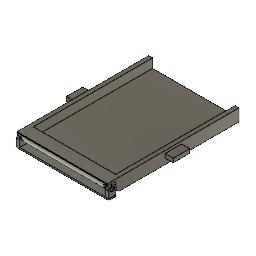
puhelimen paikka tapit ja osat v7 (Autodesk Fusion 360 design; units mm, degrees)
Autodesk Fusion 360 part; units mm, degrees
sketch "Sketch1" plane through (0, 0, 0) normal (0, 0, 1) x (1, 0, 0)
  line L0 (-50, 80) -> (60, 80)
  line L1 (60, 80) -> (60, -80)
  line L2 (60, -80) -> (-50, -80)
  line L3 (-50, -80) -> (-50, 80)
  dimension "d1" = 110
  dimension "d2" = 160
  constraint horizontal L0
  constraint vertical L1
  constraint horizontal L2
  constraint vertical L3
  measures "d1" distance of L0.start L0.end
  measures "d2" distance of L0.start L2.end
extrude "Extrude1" add sketch "Sketch1" along normal blind 12 makes body 1
sketch "Sketch2" plane through (0, 0, 12) normal (0, 0, 1) x (-1, 0, 0)
  line L0 (50, 80) -> (-60, 80)
  line L1 (-60, 80) -> (-60, -80)
  line L2 (-60, -80) -> (50, -80)
  line L3 (50, -80) -> (50, 80)
  line L4 (45, -80) -> (-55, -80)
  line L5 (-55, -80) -> (-55, 70)
  line L6 (-55, 70) -> (45, 70)
  line L7 (45, 70) -> (45, -80)
  constraint horizontal L4
  constraint vertical L5
  constraint horizontal L6
  constraint vertical L7
  constraint coincident L2 L4.start
extrude "Extrude2" cut sketch "Sketch2" against normal blind 10 contours L2 L4 L5 L6 L7 bodies 1
sketch "Sketch3" plane through (0, -70, 0) normal (0, 1, 0) x (-1, 0, 0)
  line L0 (45, 12) -> (-55, 12)
  line L1 (-55, 12) -> (-55, 2)
  line L2 (-55, 2) -> (45, 2)
  line L3 (45, 2) -> (45, 12)
  line L4 (-55, 12) -> (45, 12)
  line L5 (45, 12) -> (45, 11)
  line L6 (45, 11) -> (-55, 11)
  line L7 (-55, 11) -> (-55, 12)
  dimension "d7" = 1
  constraint horizontal L4
  constraint vertical L5
  constraint horizontal L6
  constraint vertical L7
  constraint coincident L0.end L1.start
  measures "d7" distance of L0.end L6.end
extrude "Extrude3" add sketch "Sketch3" along normal blind 5 contours L0 L1 L3 L4 L5 L6 L7 bodies 1
fillet "Fillet1" radius 12 1 edges at (5, -80, 0) on bodies 1
sketch "Sketch4" plane through (60, 0, 0) normal (1, 0, 0) x (0, 1, 0)
  arc A0 (-80, 12) -> (-68, 0) centre (-68, 12) ccw
  line L0 (-68, 0) -> (80, 0)
  line L1 (80, 0) -> (80, 12)
  line L2 (80, 12) -> (-80, 12)
  line L3 (-10, 10) -> (10, 10)
  line L4 (10, 10) -> (10, 5)
  line L5 (10, 5) -> (-10, 5)
  line L6 (-10, 5) -> (-10, 10)
  dimension "d12" = 20
  constraint horizontal L3
  constraint vertical L4
  constraint horizontal L5
  constraint vertical L6
  measures "d12" distance of L3.start L3.end
extrude "Extrude4" add sketch "Sketch4" along normal blind 10 contours L3 L4 L5 L6 bodies 1
sketch "Sketch5" plane through (-50, 0, 0) normal (-1, 0, 0) x (0, -1, 0)
  arc A0 (68, 0) -> (80, 12) centre (68, 12) ccw
  line L0 (80, 12) -> (-80, 12)
  line L1 (-80, 12) -> (-80, 0)
  line L2 (-80, 0) -> (68, 0)
  line L3 (-10, 10) -> (10, 10)
  line L4 (10, 10) -> (10, 5)
  line L5 (10, 5) -> (-10, 5)
  line L6 (-10, 5) -> (-10, 10)
  dimension "d15" = 20
  constraint horizontal L3
  constraint vertical L4
  constraint horizontal L5
  constraint vertical L6
  measures "d15" distance of L3.start L3.end
extrude "Extrude5" add sketch "Sketch5" along normal blind 10 contours L3 L4 L5 L6 bodies 1
extrude "Extrude6" add 2 faces at (-13.3333, -80, 11.9984) (21.6667, -75, 12) along direction (0, 0, 1) blind 1 on bodies 1 bodies 1
extrude "Extrude7" add 1 faces at (-13.3333, -18.6683, 0) along direction (0, 0, -1) blind 2 on bodies 1 bodies 1
fillet "Fillet2" radius 3 1 edges at (5, -68, -2) on bodies 1
sketch "Sketch6" plane through (60, 0, 0) normal (1, 0, 0) x (0, 1, 0)
  arc A0 (-68, 0) -> (-65.1716, -2) centre (-65.1716, 1) ccw
  line L0 (-65.1716, -2) -> (80, -2)
  line L1 (80, -2) -> (80, 13)
  line L2 (80, 13) -> (-80, 13)
  line L3 (-80, 13) -> (-80, 12)
  arc A1 (-80, 12) -> (-68, 0) centre (-68, 12) ccw
  line L4 (-10, 5) -> (-10, 10)
  line L5 (-10, 10) -> (10, 10)
  line L6 (10, 10) -> (10, 5)
  line L7 (10, 5) -> (-10, 5)
  line L8 (-80, 10.5) -> (-70, 10.5)
  line L9 (-70, 10.5) -> (-70, 0)
  line L10 (-70, 0) -> (-80, 0)
  line L11 (-80, 0) -> (-80, 10.5)
  dimension "d24" = 10
  constraint horizontal L8
  constraint vertical L9
  constraint horizontal L10
  constraint vertical L11
  measures "d24" distance of L8.start L8.end
extrude "Extrude8" cut sketch "Sketch6" against normal blind 5 contours A1 L8 L9 bodies 1
sketch "Sketch7" plane through (55, 0, 0) normal (1, 0, 0) x (0, 1, 0)
  arc A0 (-79.9059, 10.5) -> (-70, 0.1678) centre (-68, 12) ccw
  line L0 (-70, 0.1678) -> (-70, 2)
  line L1 (-70, 2) -> (-70, 10.5)
  line L2 (-70, 10.5) -> (-79.9059, 10.5)
  line L3 (-70, 10.5) -> (-75, 10.5)
  line L4 (-75, 10.5) -> (-75, 5.5)
  line L5 (-75, 5.5) -> (-70, 5.5)
  line L6 (-70, 5.5) -> (-70, 10.5)
  circle A1 centre (-75, 5.5) radius 2.25
  dimension "d27" = 5
  dimension "d28" = 5
  dimension "d29" = 4.5
  constraint horizontal L3
  constraint vertical L4
  constraint horizontal L5
  constraint vertical L6
  constraint coincident L1.end L2.start
  constraint coincident L4.end L5.start
  measures "d27" distance of L1.end L3.end
  measures "d28" distance of L1.end L5.end
  measures "d29" diameter of A1
extrude "Extrude9" add sketch "Sketch7" along normal blind 5 separate body contours L4 L5 A1 | L4 L5 A1 makes body 2
extrude "Extrude10" add 1 faces at (60, -73.5817, 6.0079) along direction (-1, 0, 0) blind 5 from surface at 110 on bodies 2 bodies 2 1
sketch "Sketch8" plane through (-55, 0, 0) normal (-1, 0, 0) x (0, -1, 0)
  circle A0 centre (75, 5.5) radius 2.25
  line L0 (70, 0) -> (80, 0)
  line L1 (80, 0) -> (80, 10)
  line L2 (80, 10) -> (70, 10)
  line L3 (70, 10) -> (70, 0)
  dimension "d35" = 10
  dimension "d36" = 10
  constraint horizontal L0
  constraint vertical L1
  constraint horizontal L2
  constraint vertical L3
  measures "d35" distance of L0.start L0.end
  measures "d36" distance of L0.start L2.end
extrude "Extrude11" cut sketch "Sketch8" against normal blind 10 contours A0 | L0 L1 L2 L3 bodies 1
extrude "Extrude12" add 1 faces at (60, -73.5817, 6.0079) along direction (-1, 0, 0) blind 5 from surface at 105 on bodies 2 bodies 2 1
sketch "Sketch9" plane through (-45, 0, 0) normal (-1, 0, 0) x (0, -1, 0)
  circle A0 centre (75, 5.5) radius 2.25
  arc A1 (70, 0.1678) -> (79.8322, 10) centre (68, 12) ccw
  line L0 (79.8322, 10) -> (70, 10)
  line L1 (70, 10) -> (70, 2)
  line L2 (70, 2) -> (70, 0.1678)
  line L3 (70.5, 9.5) -> (79.5, 9.5)
  line L4 (79.5, 9.5) -> (79.5, -3.5)
  line L5 (79.5, -3.5) -> (70.5, -3.5)
  line L6 (70.5, -3.5) -> (70.5, 9.5)
  dimension "d42" = 9
  dimension "d43" = 13
  constraint horizontal L3
  constraint vertical L4
  constraint horizontal L5
  constraint vertical L6
  measures "d42" distance of L3.start L3.end
  measures "d43" distance of L3.start L5.end
extrude "Extrude13" add sketch "Sketch9" along normal blind 4 from surface at 10 separate body contours A1 L3 L4 L6 | A1 L4 L5 L6 makes body 3
sketch "Sketch10" plane through (-59, 0, 0) normal (-1, 0, 0) x (0, -1, 0)
  circle A0 centre (75, 5.5) radius 2.25
  line L0 (70.5, -3.5) -> (79.5, -3.5)
  line L1 (79.5, -3.5) -> (79.5, 9.5)
  line L2 (79.5, 9.5) -> (70.5, 9.5)
  line L3 (70.5, 9.5) -> (70.5, -3.5)
  circle A1 centre (75, 5.5) radius 2.625
  dimension "d47" = 5.25
  constraint concentric A0 A1
  measures "d47" diameter of A1
extrude "Extrude14" cut sketch "Sketch10" against normal blind 5 contours A1 bodies 3
fillet "Fillet3" radius 4 2 edges at (-57, -70.5, 9.5) (-57, -79.5, 9.5) on bodies 3
copy_body "CopyPasteBodies1" bodies 3 makes body 4
sketch "Sketch11" plane through (-50, 0, 0) normal (-1, 0, 0) x (0, -1, 0)
  line L0 (70, 10) -> (79.8322, 10)
  arc A0 (79.8322, 10) -> (80, 12) centre (68, 12) ccw
  line L1 (80, 12) -> (80, 13)
  line L2 (80, 13) -> (-80, 13)
  line L3 (-80, 13) -> (-80, -2)
  line L4 (-80, -2) -> (65.1716, -2)
  arc A1 (65.1716, -2) -> (68, 0) centre (65.1716, 1) ccw
  arc A2 (68, 0) -> (70, 0.1678) centre (68, 12) ccw
  line L5 (70, 0.1678) -> (70, 10)
  line L6 (-10, 5) -> (-10, 10)
  line L7 (-10, 10) -> (10, 10)
  line L8 (10, 10) -> (10, 5)
  line L9 (10, 5) -> (-10, 5)
extrude "Extrude15" add 1 faces at (-57.6667, -76.5, -3.5) along direction (0, 0, -1) blind 0.5 on bodies 3 bodies 3 4
sketch "Sketch12" plane through (-59, 0, 0) normal (-1, 0, 0) x (0, -1, 0)
  arc A0 (79.5, 5.5) -> (75.5, 9.5) centre (75.5, 5.5) ccw
  line L0 (75.5, 9.5) -> (74.5, 9.5)
  arc A1 (74.5, 9.5) -> (70.5, 5.5) centre (74.5, 5.5) ccw
  line L1 (70.5, 5.5) -> (70.5, -4)
  line L2 (70.5, -4) -> (79.5, -4)
  line L3 (79.5, -4) -> (79.5, 5.5)
  circle A2 centre (75, 5.5) radius 2.625
extrude "Extrude16" add 1 faces at (-57.6667, -76.5, -4) along direction (0, 0, -1) blind 0.5 on bodies 3 bodies 3
sketch "Sketch13" plane through (-55, 0, 0) normal (1, 0, 0) x (0, 1, 0)
  circle A0 centre (-75, 5.5) radius 2.625
  arc A1 (-75.5, 9.5) -> (-79.5, 5.5) centre (-75.5, 5.5) ccw
  line L0 (-79.5, 5.5) -> (-79.5, -4.5)
  line L1 (-79.5, -4.5) -> (-70.5, -4.5)
  line L2 (-70.5, -4.5) -> (-70.5, 5.5)
  arc A2 (-70.5, 5.5) -> (-74.5, 9.5) centre (-74.5, 5.5) ccw
  line L3 (-74.5, 9.5) -> (-75.5, 9.5)
copy_body "CopyPasteBodies2" bodies 3 makes body 5
move_body "Move1" bodies 5 to x (1, 0, 0) y (0, 1, 0) z (0, 0, 1) at (-20, 10, 10)
extrude "Extrude17" cut 1 faces at (-77.6667, -66.5, 5.5) along direction (0, 0, 1) blind 2 on bodies 5 bodies 5
sketch "Sketch14" plane through (-55, 0, 0) normal (1, 0, 0) x (0, 1, 0)
  circle A0 centre (-75, 5.5) radius 2.625
  arc A1 (-75.5, 9.5) -> (-79.5, 5.5) centre (-75.5, 5.5) ccw
  line L0 (-79.5, 5.5) -> (-79.5, -4.5)
  line L1 (-79.5, -4.5) -> (-70.5, -4.5)
  line L2 (-70.5, -4.5) -> (-70.5, 5.5)
  arc A2 (-70.5, 5.5) -> (-74.5, 9.5) centre (-74.5, 5.5) ccw
  line L3 (-74.5, 9.5) -> (-75.5, 9.5)
  line L4 (-70.5, -4.5) -> (-79.5, -4.5)
  line L5 (-79.5, -4.5) -> (-79.5, -2.5)
  line L6 (-79.5, -2.5) -> (-70.5, -2.5)
  line L7 (-70.5, -2.5) -> (-70.5, -4.5)
  dimension "d58" = 9
  dimension "d59" = 2
  constraint horizontal L4
  constraint vertical L5
  constraint horizontal L6
  constraint vertical L7
  constraint coincident L1.end L2.start
  measures "d58" distance of L1.end L0.end
  measures "d59" distance of L1.end L6.end
extrude "Extrude18" add sketch "Sketch14" along normal blind 108 contours L0 L1 L2 L4 L5 L6 L7 bodies 3
move_body "Move2" bodies 3 to x (1, 0, 0) y (0, 1, 0) z (0, 0, 1) at (8, 0, 0)
move_body "Move3" bodies 5 to x (1, 0, 0) y (0, 1, 0) z (0, 0, 1) at (136, -10, -10)
named bodies: "pidikin", "pidikin2"
